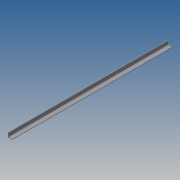
# Autodesk Inventor part: hubRingJigOuter
Saved by Autodesk Inventor 2014 SP1 (Build 180222100, 222)
## iProperties
Created: 2014-12-02
Part Number: hubRingJigOuter
Material: Generic
Document SubType Name: Modeling
Designer: Dave
Density: 1 g/cm^3
Appearance: Default
Author: Dave
Autodesk Inventor part; units mm, degrees
ref_plane "YZ Plane" through (0, 0, 0) normal (1, 0, 0) x (0, 1, 0)
ref_plane "XZ Plane" through (0, 0, 0) normal (0, 1, 0) x (-1, 0, 0)
ref_plane "XY Plane" through (0, 0, 0) normal (0, 0, 1) x (1, 0, 0)
sketch "Sketch1" plane through (0, 0, 0) normal (0, 0, 1) x (1, 0, 0)
  line L0 (0, 0) -> (0, 25.4)
  line L1 (0, 0) -> (25.4, 0)
  line L2 (3, 25.4) -> (3, 6.75)
  line L3 (6.75, 3) -> (25.4, 3)
  arc A0 (3, 6.75) -> (6.75, 3) centre (6.75, 6.75) ccw
  line L4 (0, 25.4) -> (3, 25.4)
  line L5 (25.4, 3) -> (25.4, 0)
  dimension "d0" = 25.4
  dimension "d1" = 25.4
  dimension "d2" = 3
  dimension "d3" = 3.75
  constraints: 12 end point, 3 perpendicular, 2 point on circle, 2 tangent, 1 centre point, 1 parallel, 1 vertical, 1 other
  measures "d0" distance of L0.start L0.end
  measures "d1" distance of L0.start L1.end
  measures "d2" distance between parallel lines of L2 L0
  measures "d3" radius of A0
extrude "Extrusion1" add sketch "Sketch1" along normal blind 920.4
sketch "Sketch3" plane through (6.75, 3, 0) normal (0, 1, 0) x (1, 0, 0)
  line L0 (0, 0) -> (0, -920.4) projected
  line L1 (18.65, 0) -> (18.65, -920.4) projected
  line L2 (18.65, -460.2) -> (0, -460.2) construction
  circle A0 centre (5.95, -460.2) radius 3.175
  point P0 (-6.75, 0)
  dimension "d10" = 6.35
  dimension "d11" = 12.7
  constraints: 2 end point, 2 midpoint, 1 centre point, 1 point on line
  measures "d10" diameter of A0
  measures "d11" distance from line of A0.centre L1
hole "Hole1" at (12.7, 3, 460.2) direction (0, -1, 0) diameter 6.35 end through all
equation "\"d0\" = hubAngleWidth1"
equation "\"d1\" = hubAngleWidth2"
equation "\"d2\" = hubAngleThickness"
equation "\"d3\" = 1.25 * hubAngleThickness"
equation "\"d4\" = hubOuterDiam + 2 * hubAngleThickness"
equation "\"d11\" = hubCentralHoleOffset"
equation "\"hubAngleThickness\" = 3"
equation "\"hubAngleWidth1\" = 25.4"
equation "\"hubAngleWidth2\" = 25.4"
equation "\"hubOuterDiam\" = 914.4"
equation "\"hubInnerDiam\" = 457.2"
equation "\"hubRingThickness\" = 1.524"
equation "\"hubCentralHoleOffset\" = 12.7"
body "Solid1"
